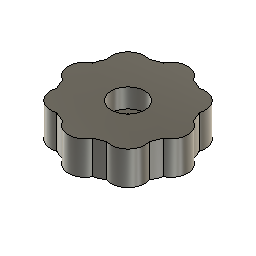
Bed Level Knob (Autodesk Fusion 360 design; units mm, degrees)
Autodesk Fusion 360 part; units mm, degrees
sketch "Sketch1" plane through (0, 0, 0) normal (0, 0, 1) x (1, 0, 0) in component "Knob"
  circle A0 centre (0, 0) radius 11
  line L0 (0, 0) -> (0, 9) construction
  arc A1 (3.1422, 10.5417) -> (-3.1422, 10.5417) centre (0, 9) ccw
  arc A2 (-5.2322, 9.6759) -> (-9.6759, 5.2322) centre (-6.364, 6.364) ccw
  arc A3 (-10.5417, 3.1422) -> (-10.5417, -3.1422) centre (-9, 0) ccw
  arc A4 (-9.6759, -5.2322) -> (-5.2322, -9.6759) centre (-6.364, -6.364) ccw
  arc A5 (-3.1422, -10.5417) -> (3.1422, -10.5417) centre (0, -9) ccw
  arc A6 (5.2322, -9.6759) -> (9.6759, -5.2322) centre (6.364, -6.364) ccw
  arc A7 (10.5417, -3.1422) -> (10.5417, 3.1422) centre (9, 0) ccw
  arc A8 (9.6759, 5.2322) -> (5.2322, 9.6759) centre (6.364, 6.364) ccw
  circle A9 centre (0, 0) radius 5.5
  circle A10 centre (0, 0) radius 2.2
  circle A11 centre (0, 0) radius 3.5
  dimension "d1" = 22
  dimension "d2" = 7
  dimension "d4" = 360
  dimension "d5" = 11
  dimension "d6" = 4.4
  dimension "d16" = 7
  constraint coincident A0.centre L0.start
  constraint vertical L0
  constraint coincident L0.end A1.centre
  constraint coincident A0 A1.start
  constraint coincident A0 A1.end
  constraint concentric A9 A10
  measures "d1" diameter of A0
  measures "d2" diameter of A1
  measures "d5" diameter of A9
  measures "d6" diameter of A10
  measures "d16" diameter of A11
extrude "Extrude1" add sketch "Sketch1" along normal blind 7 contours A0 | A0 A7 | A0 A8 | A0 A6 | A0 A1 | A0 A5 | A0 A2 | A0 A4 | A0 A3 | A9 | A11 in component "Knob"
extrude "Extrude2" add sketch "Sketch1" against normal blind 3 contours A9 | A11 in component "Knob"
extrude "Extrude3" cut sketch "Sketch1" against normal blind 4 from surface at 7 contours A11 in component "Knob"
component "Knob" placed x (1, 0, 0) y (0, 1, 0) z (0, 0, 1) at (0, 0, 0)
